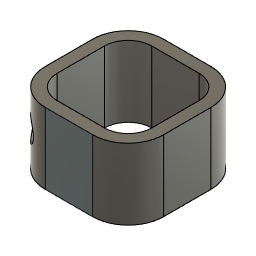
Objective_Module_Sleeve (Autodesk Fusion 360 design; units mm, degrees)
Autodesk Fusion 360 part; units mm, degrees
sketch "Sketch1" plane through (0, 0, 0) normal (0, 1, 0) x (1, 0, 0)
  line L0 (-2, -2) -> (2, -2)
  line L1 (2, -2) -> (2, 2)
  line L2 (2, 2) -> (-2, 2)
  line L3 (-2, 2) -> (-2, -2)
  line L4 (-2, -2) -> (2, 2) construction
  line L5 (2, -2) -> (-2, 2) construction
  line L6 (-2.5, -2.5) -> (2.5, -2.5)
  line L7 (2.5, -2.5) -> (2.5, 2.5)
  line L8 (2.5, 2.5) -> (-2.5, 2.5)
  line L9 (-2.5, 2.5) -> (-2.5, -2.5)
  line L10 (-2.5, -2.5) -> (2.5, 2.5) construction
  line L11 (2.5, -2.5) -> (-2.5, 2.5) construction
  dimension "d1" = 4
  dimension "d2" = 4
  dimension "d3" = 5
  dimension "d4" = 5
  constraint perpendicular L0 L1
  constraint parallel L0 L2
  constraint parallel L1 L3
  constraint horizontal L0
  constraint coincident L4 origin
  constraint coincident L5 origin
  constraint perpendicular L6 L7
  constraint parallel L6 L8
  constraint parallel L7 L9
  constraint horizontal L6
  constraint coincident L10 origin
  constraint coincident L11 origin
  measures "d1" distance of L0.end L1.end
  measures "d2" distance of L1.end L2.end
  measures "d3" distance of L7.end L8.end
  measures "d4" distance of L6.end L7.end
extrude "Extrude1" add sketch "Sketch1" along normal blind 3
fillet "Fillet1" radius 1.5 4 edges at (-2.5, 1.5, -2.5) (-2.5, 1.5, 2.5) (2.5, 1.5, -2.5) (2.5, 1.5, 2.5)
fillet "Fillet2" radius 1 4 edges at (-2, 1.5, -2) (-2, 1.5, 2) (2, 1.5, 2) (2, 1.5, -2)
sketch "Sketch2" plane through (0, 0, 2.5) normal (0, 0, 1) x (1, 0, 0)
  line L0 (1, 0) -> (1, 3)
  line L1 (1, 3) -> (-1, 3)
  line L2 (-1, 3) -> (-1, 0)
  line L3 (-1, 0) -> (1, 0)
ref_plane "WorkPlane1" through (-2.0849, 2.8811, 2.0359) normal (-0.72326, 0, 0.690576) x (-0.690576, 0, -0.72326)
sketch "Sketch3" plane through (-2.0849, 2.8811, 2.0359) normal (-0.72326, 0, 0.690576) x (-0.690576, 0, -0.72326)
  circle A0 centre (-0.0244, 1.3811) radius 0.5
  line L0 (1.0359, -0.1189) -> (-1.0849, -0.1189)
  line L1 (-1.0849, -0.1189) -> (-1.0849, 2.8811)
  line L2 (1.0359, -0.1189) -> (1.0359, 2.8811)
  dimension "d10" = 1
  dimension "d11" = 1.5
  dimension "d14" = 1.0605
  dimension "d15" = 1.097
  measures "d10" diameter of A0
  measures "d11" distance of A0.centre L0
  measures "d14" distance of A0.centre L1
extrude "Extrude2" cut sketch "Sketch3" against normal blind 0.9
